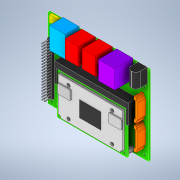
# Autodesk Inventor part: Jetson_Xavier_NX_simplified
Saved by Autodesk Inventor 2022 (Build 260153000, 153)
## iProperties
Created: 2021-09-06
Part Number: Jetson_Xavier_NX_simplified
Material: Generic
Document SubType Name: Modeling
Designer: Viktor
Density: 1 g/cm^3
Appearance: Default
Author: Viktor
Autodesk Inventor part; units mm, degrees
ref_plane "YZ Plane" through (0, 0, 0) normal (1, 0, 0) x (0, 1, 0)
ref_plane "XZ Plane" through (0, 0, 0) normal (0, 1, 0) x (-1, 0, 0)
ref_plane "XY Plane" through (0, 0, 0) normal (0, 0, 1) x (1, 0, 0)
sketch "Sketch1" plane through (0, 0, 0) normal (0, 0, 1) x (1, 0, 0)
  line L0 (-50, -39.5) -> (50, -39.5)
  line L1 (50, -39.5) -> (50, 39.5)
  line L2 (50, 39.5) -> (-50, 39.5)
  line L3 (-50, 39.5) -> (-50, -39.5)
  line L4 (-50, -39.5) -> (50, 39.5) construction
  line L5 (50, -39.5) -> (-50, 39.5) construction
  point P0 (0, 0)
  dimension "d0" = 100
  dimension "d1" = 79
  constraints: 12 end point, 2 midpoint, 2 parallel, 1 horizontal, 1 perpendicular
  measures "d0" distance of L1.end L2.end
  measures "d1" distance of L2.end L0.start
extrude "Extrusion1" add sketch "Sketch1" along normal blind 1.57
sketch "Sketch2" plane through (0, 0, 1.57) normal (0, 0, 1) x (1, 0, 0)
  circle A0 centre (-46, 22.5) radius 1.375
  circle A1 centre (-40, 22.5) radius 1.375
  circle A2 centre (46, 22.5) radius 1.375
  line L0 (-50, 39.5) -> (-50, -39.5) projected
  line L1 (50, 39.5) -> (-50, 39.5) projected
  line L2 (-46, 22.5) -> (62, 22.5) construction
  line L3 (-61, -6.5) -> (62, -6.5) construction
  line L4 (50, -39.5) -> (50, 39.5) projected
  circle A3 centre (-46, -35.5) radius 1.375
  circle A4 centre (-40, -35.5) radius 1.375
  circle A5 centre (46, -35.5) radius 1.375
  circle A6 centre (-29.8, -35.9) radius 1.375
  circle A7 centre (33.8, -35.9) radius 1.375
  line L5 (-50, -39.5) -> (50, -39.5) projected
  point P0 (0, 0)
  dimension "d4" = 6
  dimension "d5" = 2.75
  dimension "d6" = 2.75
  dimension "d7" = 2.75
  dimension "d8" = 4
  dimension "d9" = 17
  dimension "d10" = 29
  dimension "d11" = 4
  dimension "d33" = 2.75
  dimension "d34" = 2.75
  dimension "d35" = 20.2
  dimension "d36" = 16.2
  dimension "d37" = 3.6
  dimension "d38" = 3.6
  constraints: 8 centre point, 4 end point, 3 symmetric about line, 2 horizontal, 2 point on line, 3 other
  measures "d4" distance of A1.centre L2.start
  measures "d5" diameter of A0
  measures "d6" diameter of A1
  measures "d7" diameter of A2
  measures "d8" distance from line of L0 L2.start
  measures "d9" distance from line of L1 L2.start
  measures "d10" distance from line of A1.centre L3
  measures "d11" distance from line of L4 A2.centre
  measures "d33" diameter of A6
  measures "d34" diameter of A7
  measures "d35" distance from line of L0 A6.centre
  measures "d36" distance from line of L4 A7.centre
  measures "d37" distance from line of L5 A6.centre
  measures "d38" distance from line of L5 A7.centre
extrude "Extrusion2" cut sketch "Sketch2" against normal through all contours A0 | A1 | A2 | A3 | A4 | A5 | A6 | A7
fillet "Fillet1" radius 0.6 4 edges at (-50, -39.5, 0.785) (50, -39.5, 0.785) (50, 39.5, 0.785) (-50, 39.5, 0.785)
sketch "Sketch3" plane through (0, 0, 1.57) normal (0, 0, 1) x (1, 0, 0)
  line L0 (-48.54, 18.76) -> (-43.46, 18.76)
  line L1 (-43.46, 18.76) -> (-43.46, -32.04)
  line L2 (-43.46, -32.04) -> (-48.54, -32.04)
  line L3 (-48.54, -32.04) -> (-48.54, 18.76)
  line L4 (-50, 38.9) -> (-50, -38.9) projected
  line L5 (-49.4, -39.5) -> (49.4, -39.5) projected
  point P0 (0, 0)
  dimension "d15" = 1.46
  dimension "d16" = 7.46
  dimension "d17" = 5.08
  dimension "d18" = 50.8
  constraints: 8 end point, 2 parallel, 1 horizontal, 1 perpendicular
  measures "d15" distance between parallel lines of L4 L3
  measures "d16" distance between parallel lines of L5 L2
  measures "d17" distance between parallel lines of L1 L3
  measures "d18" distance between parallel lines of L2 L0
extrude "Extrusion3" add sketch "Sketch3" along normal blind 2.54 separate body
sketch "Sketch4" plane through (0, 0, 4.11) normal (0, 0, 1) x (1, 0, 0)
  line L0 (-47.59, -31.09) -> (-46.95, -31.09)
  line L1 (-46.95, -31.09) -> (-46.95, -30.45)
  line L2 (-46.95, -30.45) -> (-47.59, -30.45)
  line L3 (-47.59, -30.45) -> (-47.59, -31.09)
  line L4 (-48.54, 18.76) -> (-48.54, -32.04) projected
  line L5 (-48.54, -32.04) -> (-43.46, -32.04) projected
  point P0 (0, 0)
  dimension "d21" = 0.64
  dimension "d22" = 0.64
  dimension "d23" = 0.95
  dimension "d24" = 0.95
  constraints: 8 end point, 2 parallel, 1 horizontal, 1 perpendicular
  measures "d21" distance of L0.start L0.end
  measures "d22" distance of L2.end L0.start
  measures "d23" distance from line of L4 L0.start
  measures "d24" distance between parallel lines of L5 L0
extrude "Extrusion4" add sketch "Sketch4" along normal blind 6.06 separate body
pattern_linear "Rectangular Pattern1" count 20 spacing 2.54 along (0, 1, 0) count 2 spacing 2.54 along (1, 0, 0) of "Extrusion4" bodies 3
sketch "Sketch5" plane through (0, 0, 1.57) normal (0, 0, 1) x (1, 0, 0)
  circle A0 centre (-29.8, -35.9) radius 1.375 projected
  circle A1 centre (33.8, -35.9) radius 1.375 projected
  line L0 (-27.4906, -35.9) -> (-28.6453, -37.9)
  line L1 (-28.6453, -37.9) -> (-30.9547, -37.9)
  line L2 (-30.9547, -37.9) -> (-32.1094, -35.9)
  line L3 (-32.1094, -35.9) -> (-30.9547, -33.9)
  line L4 (-30.9547, -33.9) -> (-28.6453, -33.9)
  line L5 (-28.6453, -33.9) -> (-27.4906, -35.9)
  line L6 (36.1094, -35.9) -> (34.9547, -37.9)
  line L7 (34.9547, -37.9) -> (32.6453, -37.9)
  line L8 (32.6453, -37.9) -> (31.4906, -35.9)
  line L9 (31.4906, -35.9) -> (32.6453, -33.9)
  line L10 (32.6453, -33.9) -> (34.9547, -33.9)
  line L11 (34.9547, -33.9) -> (36.1094, -35.9)
  point P0 (0, 0)
  dimension "d39" = 4
  dimension "d40" = 4
  constraints: 24 end point, 2 coincident, 26 other
  measures "d39" distance between parallel lines of L1 L4
  measures "d40" distance between parallel lines of L7 L10
extrude "Extrusion5" add sketch "Sketch5" along normal blind 6.69 separate body
sketch "Sketch6" plane through (0, 0, 1.57) normal (0, 0, 1) x (1, 0, 0)
  line L0 (-34.5, 4.05) -> (38.5, 4.05)
  line L1 (38.5, 4.05) -> (38.5, 9.55)
  line L2 (38.5, 9.55) -> (-34.5, 9.55)
  line L3 (-34.5, 9.55) -> (-34.5, 4.05)
  line L4 (-34.5, 4.05) -> (38.5, 9.55) construction
  line L5 (38.5, 4.05) -> (-34.5, 9.55) construction
  circle A0 centre (33.8, -35.9) radius 1.375 projected
  circle A1 centre (-29.8, -35.9) radius 1.375 projected
  point P0 (0, 0)
  point P1 (2, 6.8)
  dimension "d43" = 5.5
  dimension "d44" = 73
  dimension "d45" = 63.6
  dimension "d46" = 31.8
  dimension "d47" = 45.45
  constraints: 12 end point, 2 midpoint, 2 parallel, 1 horizontal, 1 perpendicular
  measures "d43" distance between parallel lines of L0 L2
  measures "d44" distance between parallel lines of L1 L3
  measures "d45" distance of A0.centre A1.centre
  measures "d46" horizontal distance of A1.centre point (2, 6.8)
  measures "d47" distance from line of A1.centre L2
extrude "Extrusion6" add sketch "Sketch6" along normal blind 9.15 separate body contours L3 L2 L1 L0
sketch "Sketch8" plane through (0, 0, 8.26) normal (0, 0, 1) x (1, 0, 0)
  line L0 (-34.5, 4.05) -> (38.5, 4.05) projected
  line L1 (36.8, 4.05) -> (-32.8, 4.05)
  line L2 (-32.8, 4.05) -> (-32.8, -38.75)
  line L3 (-32.8, -38.75) -> (36.8, -38.75)
  line L4 (36.8, -38.75) -> (36.8, 4.05)
  line L5 (-49.4, -39.5) -> (49.4, -39.5) projected
  circle A0 centre (33.8, -35.9) radius 1.375 projected
  circle A1 centre (-29.8, -35.9) radius 1.375 projected
  point P0 (0, 0)
  point P1 (-32.8, 4.05)
  dimension "d50" = 69.6
  dimension "d51" = 0.75
  dimension "d52" = 3
  constraints: 8 end point, 2 parallel, 1 horizontal, 1 perpendicular, 1 point on line
  measures "d50" distance between parallel lines of L4 L2
  measures "d51" distance between parallel lines of L5 L3
  measures "d52" distance from line of L4 A0.centre
extrude "Extrusion7" add sketch "Sketch8" along normal blind 1.2 separate body
fillet "Fillet2" radius 0.6 2 edges at (-32.8, -38.75, 8.86) (36.8, -38.75, 8.86)
sketch "Sketch9" plane through (-34.5, 4.05, 1.57) normal (0, -1, 0) x (1, 0, 0)
  line L0 (73, 9.15) -> (0, 9.15) projected
  line L1 (0, 9.15) -> (2, 9.15)
  line L2 (2, 9.15) -> (2, 5.43)
  line L3 (2, 5.43) -> (0, 5.43)
  line L4 (0, 5.43) -> (0, 9.15)
  line L5 (2.3, 7.89) -> (70.7, 7.89) projected
  line L6 (2.3, 6.69) -> (70.7, 6.69) projected
  line L7 (36.5, 22) -> (36.5, -16) construction
  line L8 (0, 0) -> (0, 9.15) projected
  line L9 (73, 0) -> (73, 9.15) projected
  line L10 (73, 9.15) -> (71, 9.15)
  line L11 (71, 9.15) -> (71, 5.43)
  line L12 (71, 5.43) -> (73, 5.43)
  line L13 (73, 5.43) -> (73, 9.15)
  point P0 (34.5, -1.57)
  point P1 (70.7, 7.89)
  point P2 (70.7, 6.69)
  point P3 (2, 9.15)
  dimension "d56" = 1.26
  dimension "d57" = 1.26
  dimension "d58" = 2
  dimension "d59" = 36.5
  dimension "d60" = 73
  constraints: 18 end point, 5 symmetric about line, 2 parallel, 1 horizontal, 1 perpendicular, 1 vertical
  measures "d56" distance between parallel lines of L0 L5
  measures "d57" distance between parallel lines of L6 L3
  measures "d58" distance between parallel lines of L4 L2
  measures "d59" distance between parallel lines of L7 L8
  measures "d60" distance between parallel lines of L9 L8
extrude "Extrusion8" add sketch "Sketch9" along normal blind 13.7 bodies 5
sketch "Sketch10" plane through (0, 0, 9.46) normal (0, 0, 1) x (1, 0, 0)
  circle A0 centre (33.8, -35.9) radius 1.375 projected
  line L0 (-29.8, 1.35) -> (33.8, 1.35)
  line L1 (33.8, 1.35) -> (33.8, -35.9)
  line L2 (33.8, -35.9) -> (-29.8, -35.9)
  line L3 (-29.8, -35.9) -> (-29.8, 1.35)
  circle A1 centre (-29.8, -35.9) radius 1.375 projected
  circle A2 centre (-29.8, -35.9) radius 2.5
  circle A3 centre (33.8, -35.9) radius 2.5
  line L4 (-32.5, 4.05) -> (36.5, 4.05) projected
  line L5 (-32.5, 4.05) -> (-32.5, -9.65) projected
  point P0 (0, 0)
  point P1 (-29.8, -33.4)
  point P2 (-27.3, -35.9)
  point P3 (31.3, -35.9)
  point P4 (33.8, -33.4)
  dimension "d63" = 5
  dimension "d64" = 5
  dimension "d65" = 2.7
  dimension "d66" = 2.7
  constraints: 8 end point, 2 centre point, 2 parallel, 1 coincident, 1 horizontal, 1 perpendicular
  measures "d63" diameter of A2
  measures "d64" diameter of A3
  measures "d65" distance between parallel lines of L4 L0
  measures "d66" distance between parallel lines of L5 L3
extrude "Extrusion9" add sketch "Sketch10" along normal blind 2 separate body contours A3 L2 A2 L3 L0 L1
sketch "Sketch11" plane through (0, 0, 11.46) normal (0, 0, 1) x (1, 0, 0)
  line L0 (-8.8, -26.22) -> (12.8, -26.22)
  line L1 (12.8, -26.22) -> (12.8, -10.08)
  line L2 (12.8, -10.08) -> (-8.8, -10.08)
  line L3 (-8.8, -10.08) -> (-8.8, -26.22)
  line L4 (-8.8, -26.22) -> (12.8, -10.08) construction
  line L5 (12.8, -26.22) -> (-8.8, -10.08) construction
  line L6 (-32.2, -38.75) -> (36.2, -38.75) projected
  line L7 (36.8, -38.15) -> (36.8, 4.05) projected
  point P0 (0, 0)
  point P1 (2, -18.15)
  dimension "d69" = 21.6
  dimension "d70" = 16.14
  dimension "d71" = 28.67
  dimension "d72" = 24
  constraints: 12 end point, 2 midpoint, 2 parallel, 1 horizontal, 1 perpendicular
  measures "d69" distance between parallel lines of L1 L3
  measures "d70" distance between parallel lines of L0 L2
  measures "d71" distance between parallel lines of L6 L2
  measures "d72" distance between parallel lines of L7 L1
extrude "Extrusion10" add sketch "Sketch11" along normal blind 0.245 separate body
sketch "Sketch12" plane through (0, 0, 11.46) normal (0, 0, 1) x (1, 0, 0)
  line L0 (-29.45, -15.45) -> (-16.85, -15.45)
  line L1 (-16.85, -15.45) -> (-16.85, -6.05)
  line L2 (-16.85, -6.05) -> (-29.45, -6.05)
  line L3 (-29.45, -6.05) -> (-29.45, -15.45)
  line L4 (-29.45, -15.45) -> (-16.85, -6.05) construction
  line L5 (-16.85, -15.45) -> (-29.45, -6.05) construction
  line L6 (-32.8, 4.05) -> (-32.8, -38.15) projected
  line L7 (-32.2, -38.75) -> (36.2, -38.75) projected
  line L8 (2, 20) -> (2, -48) construction
  line L9 (-8.8, -10.08) -> (-8.8, -26.22) projected
  line L10 (33.45, -15.45) -> (20.85, -15.45)
  line L11 (20.85, -15.45) -> (20.85, -6.05)
  line L12 (20.85, -6.05) -> (33.45, -6.05)
  line L13 (33.45, -6.05) -> (33.45, -15.45)
  line L14 (33.45, -15.45) -> (20.85, -6.05) construction
  line L15 (20.85, -15.45) -> (33.45, -6.05) construction
  point P0 (0, 0)
  point P1 (-23.15, -10.75)
  point P2 (27.15, -10.75)
  dimension "d102" = 2.5
  dimension "d103" = 3
  dimension "d75" = 15.95
  dimension "d76" = 32.7
  dimension "d77" = 12.6
  dimension "d78" = 9.4
  dimension "d79" = 10.8
  constraints: 26 end point, 5 symmetric about line, 4 midpoint, 2 parallel, 1 horizontal, 1 perpendicular, 1 vertical
  measures "d75" distance between parallel lines of L6 L1
  measures "d76" distance between parallel lines of L7 L2
  measures "d77" distance between parallel lines of L1 L3
  measures "d78" distance between parallel lines of L0 L2
  measures "d79" distance between parallel lines of L8 L9
extrude "Extrusion11" add sketch "Sketch12" along normal blind 1 separate body
fillet "Fillet3" radius 1 8 edges at (-16.85, -15.45, 11.96) (-29.45, -15.45, 11.96) (-16.85, -6.05, 11.96) (-29.45, -6.05, 11.96) (20.85, -15.45, 11.96) (20.85, -6.05, 11.96) (33.45, -15.45, 11.96) (33.45, -6.05, 11.96)
sketch "Sketch13" plane through (0, 0, 11.46) normal (0, 0, 1) x (1, 0, 0)
  circle A0 centre (-19.6, -3.75) radius 1.6
  line L0 (-32.8, 4.05) -> (-32.8, -38.15) projected
  line L1 (-32.2, -38.75) -> (36.2, -38.75) projected
  circle A1 centre (-19.6, -32.55) radius 1.6
  line L2 (2, 15) -> (2, -44) construction
  line L3 (-8.8, -10.08) -> (-8.8, -26.22) projected
  circle A2 centre (23.6, -3.75) radius 1.6
  circle A3 centre (23.6, -32.55) radius 1.6
  point P0 (0, 0)
  dimension "d83" = 3.2
  dimension "d84" = 13.2
  dimension "d85" = 35
  dimension "d86" = 3.2
  dimension "d87" = 6.2
  dimension "d88" = 13.2
  dimension "d89" = 10.8
  constraints: 4 centre point, 2 end point, 2 symmetric about line, 1 vertical, 2 other
  measures "d83" diameter of A0
  measures "d84" distance from line of L0 A0.centre
  measures "d85" distance from line of L1 A0.centre
  measures "d86" diameter of A1
  measures "d87" distance from line of L1 A1.centre
  measures "d88" distance from line of L0 A1.centre
  measures "d89" distance between parallel lines of L3 L2
extrude "Extrusion12" cut sketch "Sketch13" against normal through all bodies 7 6
sketch "Sketch14" plane through (0, 0, 1.57) normal (0, 0, 1) x (1, 0, 0)
  line L0 (42.95, -30.2) -> (46.85, -30.2)
  line L1 (46.85, -30.2) -> (46.85, -7.8)
  line L2 (46.85, -7.8) -> (42.95, -7.8)
  line L3 (42.95, -7.8) -> (42.95, -30.2)
  line L4 (42.95, -30.2) -> (46.85, -7.8) construction
  line L5 (46.85, -30.2) -> (42.95, -7.8) construction
  line L6 (42.95, -5.2) -> (46.85, -5.2)
  line L7 (46.85, -5.2) -> (46.85, 17.2)
  line L8 (46.85, 17.2) -> (42.95, 17.2)
  line L9 (42.95, 17.2) -> (42.95, -5.2)
  line L10 (42.95, -5.2) -> (46.85, 17.2) construction
  line L11 (46.85, -5.2) -> (42.95, 17.2) construction
  line L12 (-49.4, -39.5) -> (49.4, -39.5) projected
  line L13 (50, -38.9) -> (50, 38.9) projected
  point P0 (0, 0)
  point P1 (44.9, -19)
  point P2 (44.9, 6)
  dimension "d92" = 22.4
  dimension "d93" = 22.4
  dimension "d94" = 3.9
  dimension "d95" = 3.9
  dimension "d96" = 2.6
  dimension "d97" = 9.3
  dimension "d98" = 3.15
  constraints: 24 end point, 4 midpoint, 4 parallel, 2 horizontal, 2 perpendicular, 1 point on line
  measures "d92" distance between parallel lines of L0 L2
  measures "d93" distance between parallel lines of L6 L8
  measures "d94" distance between parallel lines of L1 L3
  measures "d95" distance between parallel lines of L7 L9
  measures "d96" distance between parallel lines of L2 L6
  measures "d97" distance between parallel lines of L12 L0
  measures "d98" distance between parallel lines of L13 L1
extrude "Extrusion13" add sketch "Sketch14" along normal blind 7.776 separate body
sketch "Sketch15" plane through (0, 0, 9.346) normal (0, 0, 1) x (1, 0, 0)
  line L0 (42.95, -7.8) -> (42.95, -30.2) projected
  line L1 (42.95, 17.2) -> (42.95, -5.2) projected
  line L2 (42.95, -7.8) -> (42.95, -30.2) projected
  line L3 (42.95, -10.8) -> (44.35, -10.8)
  line L4 (44.35, -10.8) -> (44.35, -27.2)
  line L5 (44.35, -27.2) -> (42.95, -27.2)
  line L6 (42.95, -27.2) -> (42.95, -10.8)
  line L7 (42.95, 14.2) -> (44.35, 14.2)
  line L8 (44.35, 14.2) -> (44.35, -2.2)
  line L9 (44.35, -2.2) -> (42.95, -2.2)
  line L10 (42.95, -2.2) -> (42.95, 14.2)
  line L11 (46.85, -5.2) -> (46.85, 17.2) projected
  line L12 (46.85, -30.2) -> (46.85, -7.8) projected
  line L13 (46.85, -7.8) -> (42.95, -7.8) projected
  line L14 (42.95, -30.2) -> (46.85, -30.2) projected
  line L15 (42.95, -5.2) -> (46.85, -5.2) projected
  line L16 (46.85, 17.2) -> (42.95, 17.2) projected
  point P0 (0, 0)
  dimension "d101" = 2.5
  dimension "d102" = 2.5
  dimension "d103" = 3
  dimension "d104" = 3
  dimension "d105" = 3
  dimension "d106" = 3
  constraints: 16 end point, 4 parallel, 3 point on line, 2 horizontal, 2 perpendicular
  measures "d101" distance between parallel lines of L11 L8
  measures "d102" distance between parallel lines of L12 L4
  measures "d103" distance between parallel lines of L13 L3
  measures "d104" distance between parallel lines of L14 L5
  measures "d105" distance between parallel lines of L15 L9
  measures "d106" distance between parallel lines of L16 L7
extrude "Extrusion14" cut sketch "Sketch15" against normal blind 3 contours L3 L4 L5 L0 | L7 L8 L9 L1 bodies 10
sketch "Sketch16" plane through (0, 0, 9.346) normal (0, 0, 1) x (1, 0, 0)
  line L0 (46.85, 17.2) -> (42.95, 17.2) projected
  line L1 (46.85, -5.2) -> (46.85, 17.2) projected
  line L2 (42.95, -5.2) -> (46.85, -5.2) projected
  line L3 (45.35, -5.2) -> (45.35, -3.3422)
  line L4 (45.35, -3.3422) -> (46.85, -1.2)
  line L5 (46.85, -5.2) -> (46.85, 17.2) projected
  line L6 (45.35, 17.2) -> (45.35, 15.3422)
  line L7 (45.35, 15.3422) -> (46.85, 13.2)
  line L8 (41, -6.5) -> (68, -6.5) construction
  line L9 (46.85, -7.8) -> (42.95, -7.8) projected
  line L10 (45.35, -7.8) -> (45.35, -9.6578)
  line L11 (45.35, -9.6578) -> (46.85, -11.8)
  line L12 (45.35, -30.2) -> (45.35, -28.3422)
  line L13 (45.35, -28.3422) -> (46.85, -26.2)
  line L14 (46.85, -30.2) -> (46.85, -7.8) projected
  line L15 (42.95, -30.2) -> (46.85, -30.2) projected
  line L16 (45.35, -7.8) -> (46.85, -7.8)
  line L17 (46.85, -11.8) -> (46.85, -7.8)
  line L18 (45.35, -30.2) -> (46.85, -30.2)
  line L19 (46.85, -26.2) -> (46.85, -30.2)
  line L20 (45.35, -5.2) -> (46.85, -5.2)
  line L21 (46.85, -5.2) -> (46.85, -1.2)
  line L22 (46.85, 13.2) -> (46.85, 17.2)
  line L23 (46.85, 17.2) -> (45.35, 17.2)
  point P0 (0, 0)
  dimension "d109" = 145
  dimension "d110" = 145
  dimension "d111" = 4
  dimension "d112" = 4
  dimension "d113" = 1.5
  dimension "d114" = 2.6
  dimension "d115" = 1.3
  constraints: 34 end point, 8 point on line, 6 symmetric about line, 3 collinear, 2 perpendicular, 1 horizontal, 1 vertical
  measures "d109" angle of L6 L7
  measures "d110" angle of L4 L3
  measures "d111" distance from line of L2 L4.end
  measures "d112" distance from line of L0 L7.end
  measures "d113" distance between parallel lines of L1 L6
  measures "d114" distance from line of L9 L2.start
  measures "d115" distance between parallel lines of L8 L2
extrude "Extrusion15" cut sketch "Sketch16" against normal up to surface (7.776 mm away) bodies 10
sketch "Sketch17" plane through (0, 0, 1.57) normal (0, 0, 1) x (1, 0, 0)
  line L0 (-46, 40.1) -> (-38, 40.1)
  line L1 (-38, 40.1) -> (-38, 33.5)
  line L2 (-38, 33.5) -> (-46, 33.5)
  line L3 (-46, 33.5) -> (-46, 40.1)
  line L4 (-46, 40.1) -> (-38, 33.5) construction
  line L5 (-38, 40.1) -> (-46, 33.5) construction
  line L6 (49.4, 39.5) -> (-49.4, 39.5) projected
  line L7 (-50, 38.9) -> (-50, -38.9) projected
  point P0 (0, 0)
  point P1 (-42, 36.8)
  point P2 (-38, 39.5)
  point P3 (-46, 39.5)
  dimension "d118" = 8
  dimension "d119" = 6.6
  dimension "d120" = 6
  dimension "d121" = 4
  constraints: 12 end point, 2 midpoint, 2 parallel, 1 horizontal, 1 perpendicular
  measures "d118" distance of L0.start L0.end
  measures "d119" distance between parallel lines of L2 L0
  measures "d120" distance between parallel lines of L6 L2
  measures "d121" distance between parallel lines of L7 L3
extrude "Extrusion16" add sketch "Sketch17" along normal blind 2.7 separate body
sketch "Sketch18" plane through (0, 0, 1.57) normal (0, 0, 1) x (1, 0, 0)
  line L0 (-34.9, 20.65) -> (-19, 20.65)
  line L1 (-19, 20.65) -> (-19, 42)
  line L2 (-19, 42) -> (-34.9, 42)
  line L3 (-34.9, 42) -> (-34.9, 20.65)
  line L4 (-34.9, 20.65) -> (-19, 42) construction
  line L5 (-19, 20.65) -> (-34.9, 42) construction
  line L6 (-50, 38.9) -> (-50, -38.9) projected
  line L7 (49.4, 39.5) -> (-49.4, 39.5) projected
  point P0 (0, 0)
  point P1 (-26.95, 31.325)
  dimension "d124" = 15.1
  dimension "d125" = 18.85
  dimension "d126" = 21.35
  dimension "d127" = 15.9
  constraints: 12 end point, 2 midpoint, 2 parallel, 1 horizontal, 1 perpendicular
  measures "d124" distance between parallel lines of L6 L3
  measures "d125" distance between parallel lines of L7 L0
  measures "d126" distance between parallel lines of L2 L0
  measures "d127" distance between parallel lines of L1 L3
extrude "Extrusion17" add sketch "Sketch18" along normal blind 13.65 separate body
sketch "Sketch19" plane through (0, 0, 1.57) normal (0, 0, 1) x (1, 0, 0)
  line L0 (-16.475, 23.75) -> (-2.825, 23.75)
  line L1 (-2.825, 23.75) -> (-2.825, 41.15)
  line L2 (-2.825, 41.15) -> (-16.475, 41.15)
  line L3 (-16.475, 41.15) -> (-16.475, 23.75)
  line L4 (-16.475, 23.75) -> (-2.825, 41.15) construction
  line L5 (-2.825, 23.75) -> (-16.475, 41.15) construction
  line L6 (-50, 38.9) -> (-50, -38.9) projected
  line L7 (49.4, 39.5) -> (-49.4, 39.5) projected
  line L8 (-1.2, 44) -> (-1.2, 20) construction
  line L9 (14.075, 23.75) -> (0.425, 23.75)
  line L10 (0.425, 23.75) -> (0.425, 41.15)
  line L11 (0.425, 41.15) -> (14.075, 41.15)
  line L12 (14.075, 41.15) -> (14.075, 23.75)
  line L13 (14.075, 23.75) -> (0.425, 41.15) construction
  line L14 (0.425, 23.75) -> (14.075, 41.15) construction
  point P0 (0, 0)
  point P1 (-9.65, 32.45)
  point P2 (7.25, 32.45)
  point P3 (14.075, 39.5)
  point P4 (0.425, 39.5)
  point P5 (-2.825, 39.5)
  point P6 (-16.475, 39.5)
  dimension "d130" = 13.65
  dimension "d131" = 17.4
  dimension "d132" = 33.525
  dimension "d133" = 15.75
  dimension "d134" = 1.625
  constraints: 26 end point, 5 symmetric about line, 4 midpoint, 2 parallel, 1 horizontal, 1 perpendicular, 1 vertical
  measures "d130" distance between parallel lines of L1 L3
  measures "d131" distance between parallel lines of L0 L2
  measures "d132" distance between parallel lines of L6 L3
  measures "d133" distance between parallel lines of L7 L0
  measures "d134" distance between parallel lines of L1 L8
extrude "Extrusion18" add sketch "Sketch19" along normal blind 16.566 separate body
sketch "Sketch20" plane through (0, 0, 1.57) normal (0, 0, 1) x (1, 0, 0)
  line L0 (18.225, 23.275) -> (34.285, 23.275)
  line L1 (34.285, 23.275) -> (34.285, 41.525)
  line L2 (34.285, 41.525) -> (18.225, 41.525)
  line L3 (18.225, 41.525) -> (18.225, 23.275)
  line L4 (18.225, 23.275) -> (34.285, 41.525) construction
  line L5 (34.285, 23.275) -> (18.225, 41.525) construction
  line L6 (50, -38.9) -> (50, 38.9) projected
  line L7 (49.4, 39.5) -> (-49.4, 39.5) projected
  point P0 (0, 0)
  point P1 (26.255, 32.4)
  dimension "d137" = 16.06
  dimension "d138" = 18.25
  dimension "d139" = 15.715
  dimension "d140" = 16.225
  constraints: 12 end point, 2 midpoint, 2 parallel, 1 horizontal, 1 perpendicular
  measures "d137" distance between parallel lines of L1 L3
  measures "d138" distance between parallel lines of L0 L2
  measures "d139" distance between parallel lines of L6 L1
  measures "d140" distance between parallel lines of L7 L0
extrude "Extrusion19" add sketch "Sketch20" along normal blind 18.176 separate body
sketch "Sketch21" plane through (0, 0, 1.57) normal (0, 0, 1) x (1, 0, 0)
  line L0 (39.5, 26.6) -> (48.5, 26.6)
  line L1 (48.5, 26.6) -> (48.5, 41)
  line L2 (48.5, 41) -> (39.5, 41)
  line L3 (39.5, 41) -> (39.5, 26.6)
  line L4 (39.5, 26.6) -> (48.5, 41) construction
  line L5 (48.5, 26.6) -> (39.5, 41) construction
  line L6 (50, -38.9) -> (50, 38.9) projected
  line L7 (49.4, 39.5) -> (-49.4, 39.5) projected
  point P0 (0, 0)
  point P1 (44, 33.8)
  dimension "d143" = 9
  dimension "d144" = 14.4
  dimension "d145" = 1.5
  dimension "d148" = 12.9
  constraints: 12 end point, 2 midpoint, 2 parallel, 1 horizontal, 1 perpendicular
  measures "d143" distance between parallel lines of L1 L3
  measures "d144" distance between parallel lines of L2 L0
  measures "d145" distance between parallel lines of L6 L1
  measures "d148" distance between parallel lines of L7 L0
extrude "Extrusion20" add sketch "Sketch21" along normal blind 11.4 separate body
fillet "Fillet4" radius 4.25 2 edges at (39.5, 33.8, 12.97) (48.5, 33.8, 12.97)
equation "\"d6\" = d5"
equation "\"d7\" = d5"
equation "\"d11\" = d8"
equation "\"d34\" = d33"
equation "\"d38\" = d37"
equation "\"d40\" = d39"
equation "\"d46\" = 0.5 * d45"
equation "\"d57\" = d56"
equation "\"d59\" = 0.5 * d60"
equation "\"d64\" = d63"
equation "\"d65\" = d66"
equation "\"d93\" = d92"
equation "\"d95\" = d94"
equation "\"d105\" = d104"
equation "\"d106\" = d105"
equation "\"d110\" = d109"
equation "\"d112\" = d111"
body "Solid1"
body "Solid2"
body "Solid3"
body "Solid4"
body "Solid5"
body "Solid6"
body "Solid8"
body "Solid9"
body "Solid10"
